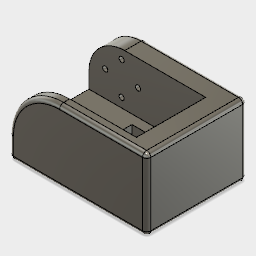
top_bracket (Autodesk Fusion 360 design; units mm, degrees)
Autodesk Fusion 360 part; units mm, degrees
sketch "Sketch1" plane through (0, 0, 0) normal (0, 1, 0) x (1, 0, 0)
  line L0 (0, 0) -> (50, 0)
  line L1 (50, 0) -> (50, -31.77)
  line L2 (50, -31.77) -> (0, -31.77)
  line L3 (0, -31.77) -> (0, 0)
  line L4 (0, 0) -> (0, -15.885)
  line L5 (0, -15.885) -> (0, -9.635)
  line L6 (0, -15.885) -> (0, -22.135)
  line L7 (0, -22.135) -> (3.4, -22.135)
  line L8 (0, -9.635) -> (3.4, -9.635)
  circle A0 centre (3.4, -9.635) radius 1
  circle A1 centre (3.4, -22.135) radius 1
  line L9 (0, -15.885) -> (0, -7.885)
  line L10 (0, -15.885) -> (0, -23.885)
  line L11 (0, -7.885) -> (17, -7.885)
  line L12 (0, -23.885) -> (17, -23.885)
  circle A2 centre (17, -23.885) radius 1
  circle A3 centre (17, -7.885) radius 1
  line L13 (0, -15.885) -> (10.8, -15.885)
  circle A4 centre (10.8, -15.885) radius 5.375
  line L14 (0, -23.885) -> (33, -23.885)
  line L15 (0, -7.885) -> (33, -7.885)
  circle A5 centre (33, -7.885) radius 1
  circle A6 centre (33, -23.885) radius 1
  line L16 (0, -15.885) -> (43.5, -15.885)
  line L17 (43.5, -15.885) -> (43.5, -25.885)
  line L18 (43.5, -15.885) -> (43.5, -5.885)
  line L19 (43.5, -5.885) -> (36.36, -5.885)
  line L20 (43.5, -25.885) -> (36.36, -25.885)
  line L21 (36.36, -25.885) -> (36.36, -19.885)
  line L22 (36.36, -5.885) -> (36.36, -11.885)
  line L23 (36.36, -11.885) -> (43.5, -11.885)
  line L24 (36.36, -19.885) -> (43.5, -19.885)
  line L25 (0, -15.885) -> (24, -15.885)
  line L26 (24, -15.885) -> (31, -15.885)
  line L27 (31, -15.885) -> (31.5, -15.885)
  line L28 (24, -15.885) -> (24, -3.885)
  line L29 (31.5, -15.885) -> (31.5, -3.885)
  line L30 (31.5, -15.885) -> (31.5, -27.885)
  line L31 (24, -15.885) -> (24, -27.885)
  line L32 (31.5, -3.885) -> (24, -3.885)
  line L33 (24, -27.885) -> (31.5, -27.885)
  line L34 (24, -27.885) -> (22, -27.885)
  line L35 (22, -27.885) -> (22, -3.885)
  line L36 (22, -3.885) -> (24, -3.885)
  dimension "d1" = 50
  dimension "d2" = 31.77
  dimension "d3" = 6.25
  dimension "d4" = 6.25
  dimension "d5" = 3.4
  dimension "d6" = 3.4
  dimension "d7" = 2
  dimension "d8" = 2
  dimension "d9" = 8
  dimension "d10" = 8
  dimension "d11" = 17
  dimension "d12" = 17
  dimension "d13" = 2
  dimension "d14" = 2
  dimension "d15" = 10.8
  dimension "d16" = 10.75
  dimension "d17" = 33
  dimension "d18" = 33
  dimension "d19" = 2
  dimension "d20" = 2
  dimension "d21" = 43.5
  dimension "d22" = 10
  dimension "d23" = 10
  dimension "d24" = 7.14
  dimension "d25" = 7.14
  dimension "d26" = 6
  dimension "d27" = 6
  dimension "d28" = 24
  dimension "d29" = 7
  dimension "d30" = 0.5
  dimension "d31" = 12
  dimension "d32" = 12
  dimension "d33" = 12
  dimension "d34" = 12
  dimension "d35" = 2
  dimension "d36" = 24
  constraint horizontal L0
  constraint vertical L1
  constraint horizontal L2
  constraint vertical L3
  constraint coincident L0.start L3.end
  constraint midpoint L3
  constraint horizontal L11
  constraint vertical L17
  constraint vertical L18
  constraint vertical L22
  constraint coincident L18
  constraint perpendicular L18 L23
  constraint coincident L17 L0.start
  constraint perpendicular L17 L24
  constraint perpendicular L28 L32
  constraint perpendicular L30 L33
  constraint perpendicular L31 L34
  constraint perpendicular L28 L36
  measures "d2" distance of L0.start
  measures "d3" distance of L0.start
  measures "d7" diameter of A0
  measures "d8" diameter of A1
  measures "d9" distance of L0.start
  measures "d13" diameter of A2
  measures "d14" diameter of A3
  measures "d16" diameter of A4
  measures "d19" diameter of A5
  measures "d20" diameter of A6
  measures "d23" distance of L0.start
  measures "d26" distance of L0.start
  measures "d27" distance of L0.start
  measures "d33" distance of L0.start
  measures "d34" distance of L0.start
  measures "d36" distance of L0.start
extrude "Extrude1" add sketch "Sketch1" along normal blind 3 contours L0 L1 L2 L3 L4 L11 L12 A2 A3 L14 L15 L29 L30 L32 L33 L34 L35 L36 | L3 L4 L5 L9 L11 A3 L13 A4 L15 L16 L25 L35 | L3 L6 L10 L12 A2 L13 A4 L14 L16 L25 L35
extrude "Extrude2" add sketch "Sketch1" along normal blind 7 contours L13 A4 L16 L25 | L13 A4 L16 L25 | L17 L20 L21 L24 | L18 L19 L22 L23
extrude "Extrude3" add 1 faces at (44.6337, 0, 13.363) along direction (0, -1, 0) blind 7
extrude "Extrude4" cut 3 faces at (38.74, 7, 21.885) (41.12, 7, 9.885) (11.9171, 7, 13.428) along direction (0, -1, 0) blind 8
sketch "Sketch2" plane through (0, 3, 0) normal (0, 1, 0) x (-1, 0, 0)
  circle A0 centre (-33, 7.885) radius 1
  line L0 (-43.5, 11.885) -> (-36.36, 11.885)
  line L1 (-36.36, 11.885) -> (-36.36, 5.885)
  line L2 (-36.36, 5.885) -> (-43.5, 5.885)
  line L3 (-43.5, 5.885) -> (-43.5, 11.885)
  circle A1 centre (-33, 23.885) radius 1
  line L4 (-36.36, 25.885) -> (-36.36, 19.885)
  line L5 (-36.36, 19.885) -> (-43.5, 19.885)
  line L6 (-43.5, 19.885) -> (-43.5, 25.885)
  line L7 (-43.5, 25.885) -> (-36.36, 25.885)
  circle A2 centre (-3.4, 22.135) radius 1
  circle A3 centre (-17, 23.885) radius 1
  circle A4 centre (-17, 7.885) radius 1
  circle A5 centre (-3.4, 9.635) radius 1
  circle A6 centre (-10.8, 15.885) radius 5.375
  line L8 (-31.5, 27.885) -> (-22, 27.885)
  line L9 (-22, 27.885) -> (-22, 3.885)
  line L10 (-22, 3.885) -> (-31.5, 3.885)
  line L11 (-31.5, 3.885) -> (-31.5, 27.885)
  line L12 (0, 0) -> (0, 31.77)
  line L13 (0, 31.77) -> (-50, 31.77)
  line L14 (-50, 31.77) -> (-50, 0)
  line L15 (-50, 0) -> (0, 0)
  line L16 (-20.4906, 2.4501) -> (-32.562, 2.4501)
  line L17 (-32.562, 2.4501) -> (-32.562, 29.6236)
  line L18 (-32.562, 29.6236) -> (-20.4906, 29.6236)
  line L19 (-20.4906, 29.6236) -> (-20.4906, 2.4501)
  circle A7 centre (-10.8, 15.885) radius 5.75
  line L20 (-36, 5.5) -> (-44, 5.5)
  line L21 (-44, 5.5) -> (-44, 12.5)
  line L22 (-44, 12.5) -> (-36, 12.5)
  line L23 (-36, 12.5) -> (-36, 5.5)
  line L24 (-36, 19.5) -> (-43.8348, 19.5)
  line L25 (-43.8348, 19.5) -> (-43.8348, 26.2715)
  line L26 (-43.8348, 26.2715) -> (-36, 26.2715)
  line L27 (-36, 26.2715) -> (-36, 19.5)
  circle A8 centre (-33, 23.885) radius 1.25
  circle A9 centre (-33, 7.885) radius 1.25
  circle A10 centre (-17, 7.885) radius 1.25
  circle A11 centre (-17, 23.885) radius 1.25
  circle A12 centre (-3.4, 22.135) radius 1.25
  circle A13 centre (-3.4, 9.635) radius 1.25
  dimension "d45" = 11.5
  dimension "d46" = 2.5
  dimension "d47" = 2.5
  dimension "d48" = 2.5
  dimension "d49" = 2.5
  dimension "d50" = 2.5
  dimension "d51" = 2.5
  constraint horizontal L16
  constraint vertical L17
  constraint horizontal L18
  constraint vertical L19
  constraint concentric A6 A7
  constraint horizontal L20
  constraint vertical L21
  constraint horizontal L22
  constraint vertical L23
  constraint horizontal L24
  constraint vertical L25
  constraint horizontal L26
  constraint vertical L27
  constraint concentric A1 A8
  constraint concentric A0 A9
  constraint concentric A4 A10
  constraint concentric A3 A11
  constraint concentric A2 A12
  constraint concentric A5 A13
  measures "d45" diameter of A7
  measures "d46" diameter of A8
  measures "d47" diameter of A9
  measures "d48" diameter of A10
  measures "d49" diameter of A11
  measures "d50" diameter of A12
  measures "d51" diameter of A13
extrude "Extrude5" cut sketch "Sketch2" against normal blind 4 contours A7 | L20 L21 L22 L23 | L24 L25 L26 L27
extrude "Extrude6" cut sketch "Sketch2" against normal blind 11 contours A0 L17 A9 | A0 L17 A9 | L16 L17 L18 L19 A8 A9 | A1 L17 A8 | A1 L17 A8 | A10 | A11 | A12 | A13
extrude "Extrude7" add 1 faces at (16.6667, -0.3333, 0) along direction (0, 0, -1) blind 12
sketch "Sketch3" plane through (0, 3, 0) normal (0, 1, 0) x (-1, 0, 0)
  circle A0 centre (-3.4, 9.635) radius 1.25
  circle A1 centre (-17, 7.885) radius 1.25
  circle A2 centre (-3.4, 22.135) radius 1.25
  circle A3 centre (-17, 23.885) radius 1.25
  line L0 (-32.562, 9.0557) -> (-32.562, 22.7143)
  arc A4 (-32.562, 25.0557) -> (-32.562, 22.7143) centre (-33, 23.885) ccw
  line L1 (-32.562, 25.0557) -> (-32.562, 29.6236)
  line L2 (-32.562, 29.6236) -> (-20.4906, 29.6236)
  line L3 (-20.4906, 29.6236) -> (-20.4906, 2.4501)
  line L4 (-20.4906, 2.4501) -> (-32.562, 2.4501)
  line L5 (-32.562, 2.4501) -> (-32.562, 6.7143)
  arc A5 (-32.562, 9.0557) -> (-32.562, 6.7143) centre (-33, 7.885) ccw
  circle A6 centre (-10.8, 15.885) radius 5.75
  line L6 (-44, 5.5) -> (-44, 12.5)
  line L7 (-44, 12.5) -> (-36, 12.5)
  line L8 (-36, 12.5) -> (-36, 5.5)
  line L9 (-36, 5.5) -> (-44, 5.5)
  line L10 (-43.8348, 19.5) -> (-43.8348, 26.2715)
  line L11 (-43.8348, 26.2715) -> (-36, 26.2715)
  line L12 (-36, 26.2715) -> (-36, 19.5)
  line L13 (-36, 19.5) -> (-43.8348, 19.5)
  line L14 (0, -12) -> (0, 31.77)
  line L15 (0, 31.77) -> (-50, 31.77)
  line L16 (-50, 31.77) -> (-50, -12)
  line L17 (-50, -12) -> (0, -12)
  line L18 (0, -12) -> (-50, -12)
  line L19 (-50, -12) -> (-50, -2)
  line L20 (-50, -2) -> (0, -2)
  line L21 (0, -2) -> (0, -12)
  dimension "d58" = 10
  constraint horizontal L18
  constraint vertical L19
  constraint horizontal L20
  constraint vertical L21
extrude "Extrude8" add sketch "Sketch3" along normal blind 25 contours L14 L16 L17 L18 L19 L20 L21
extrude "Extrude9" add 1 faces at (50, -3.6667, 5.9233) along direction (1, 0, 0) blind 12
sketch "Sketch4" plane through (0, 3, 0) normal (0, 1, 0) x (-1, 0, 0)
  line L0 (-62, -2) -> (0, -2)
  line L1 (0, -2) -> (0, 31.77)
  line L2 (0, 31.77) -> (-62, 31.77)
  line L3 (-62, 31.77) -> (-62, -2)
  line L4 (-43.8348, 19.5) -> (-43.8348, 26.2715)
  line L5 (-43.8348, 26.2715) -> (-36, 26.2715)
  line L6 (-36, 26.2715) -> (-36, 19.5)
  line L7 (-36, 19.5) -> (-43.8348, 19.5)
  line L8 (-44, 5.5) -> (-44, 12.5)
  line L9 (-44, 12.5) -> (-36, 12.5)
  line L10 (-36, 12.5) -> (-36, 5.5)
  line L11 (-36, 5.5) -> (-44, 5.5)
  circle A0 centre (-10.8, 15.885) radius 5.75
  line L12 (-32.562, 9.0557) -> (-32.562, 22.7143)
  arc A1 (-32.562, 25.0557) -> (-32.562, 22.7143) centre (-33, 23.885) ccw
  line L13 (-32.562, 25.0557) -> (-32.562, 29.6236)
  line L14 (-32.562, 29.6236) -> (-20.4906, 29.6236)
  line L15 (-20.4906, 29.6236) -> (-20.4906, 2.4501)
  line L16 (-20.4906, 2.4501) -> (-32.562, 2.4501)
  line L17 (-32.562, 2.4501) -> (-32.562, 6.7143)
  arc A2 (-32.562, 9.0557) -> (-32.562, 6.7143) centre (-33, 7.885) ccw
  circle A3 centre (-17, 23.885) radius 1.25
  circle A4 centre (-3.4, 22.135) radius 1.25
  circle A5 centre (-17, 7.885) radius 1.25
  circle A6 centre (-3.4, 9.635) radius 1.25
  line L18 (-62, 31.77) -> (-52, 31.77)
  line L19 (-52, 31.77) -> (-52, -2)
  line L20 (-52, -2) -> (-62, -2)
  line L21 (-62, -2) -> (-62, 31.77)
  dimension "d63" = 10
  constraint horizontal L18
  constraint vertical L19
  constraint horizontal L20
  constraint vertical L21
extrude "Extrude10" add sketch "Sketch4" along normal blind 25 contours L0 L2 L3 L18 L19 L20 L21
sketch "Sketch5" plane through (0, 0, -2) normal (0, 0, 1) x (1, 0, 0)
  line L0 (52, 3) -> (52, 28)
  line L1 (52, 28) -> (0, 28)
  line L2 (0, 28) -> (0, 3)
  line L3 (0, 3) -> (52, 3)
  line L4 (0, 28) -> (3, 28)
  line L5 (3, 28) -> (3, 15.5)
  line L6 (3, 15.5) -> (11, 15.5)
  line L7 (11, 15.5) -> (11, 23.5)
  line L8 (11, 15.5) -> (11, 7.5)
  line L9 (11, 15.5) -> (19, 15.5)
  circle A0 centre (19, 15.5) radius 1.25
  circle A1 centre (11, 23.5) radius 1.25
  circle A2 centre (11, 7.5) radius 1.25
  circle A3 centre (3, 15.5) radius 1.25
  dimension "d66" = 3
  dimension "d67" = 12.5
  dimension "d68" = 8
  dimension "d69" = 8
  dimension "d70" = 8
  dimension "d71" = 8
  dimension "d72" = 2.5
  dimension "d73" = 2.5
  dimension "d74" = 2.5
  dimension "d75" = 2.5
  constraint coincident L1
  constraint perpendicular L2 L4
  constraint perpendicular L5 L6
  measures "d72" diameter of A0
  measures "d73" diameter of A1
  measures "d74" diameter of A2
  measures "d75" diameter of A3
extrude "Extrude11" cut sketch "Sketch5" against normal blind 23 contours L5 L6 A3 | L5 L6 A3 | A0 | A1 | A2
extrude "Extrude12" cut 1 faces at (52.7454, -7, 9.2799) along direction (0, 1, 0) blind 6
sketch "Sketch6" plane through (0, -1, 0) normal (0, -1, 0) x (1, 0, 0)
  circle A0 centre (10.8, 15.885) radius 5.75
  line L0 (44, 12.5) -> (44, 5.5)
  line L1 (44, 5.5) -> (36, 5.5)
  line L2 (36, 5.5) -> (36, 12.5)
  line L3 (36, 12.5) -> (44, 12.5)
  line L4 (43.8348, 26.2715) -> (43.8348, 19.5)
  line L5 (43.8348, 19.5) -> (36, 19.5)
  line L6 (36, 19.5) -> (36, 26.2715)
  line L7 (36, 26.2715) -> (43.8348, 26.2715)
  circle A1 centre (3.4, 9.635) radius 1.25
  circle A2 centre (17, 7.885) radius 1.25
  circle A3 centre (3.4, 22.135) radius 1.25
  circle A4 centre (17, 23.885) radius 1.25
  line L8 (32.562, 22.7143) -> (32.562, 9.0557)
  arc A5 (32.562, 6.7143) -> (32.562, 9.0557) centre (33, 7.885) ccw
  line L9 (32.562, 6.7143) -> (32.562, 2.4501)
  line L10 (32.562, 2.4501) -> (20.4906, 2.4501)
  line L11 (20.4906, 2.4501) -> (20.4906, 29.6236)
  line L12 (20.4906, 29.6236) -> (32.562, 29.6236)
  line L13 (32.562, 29.6236) -> (32.562, 25.0557)
  arc A6 (32.562, 22.7143) -> (32.562, 25.0557) centre (33, 23.885) ccw
  line L14 (0, 31.77) -> (0, -12)
  line L15 (0, -12) -> (62, -12)
  line L16 (62, -12) -> (62, 31.77)
  line L17 (62, 31.77) -> (0, 31.77)
  circle A7 centre (3.4, 9.635) radius 2.5
  circle A8 centre (3.4, 22.135) radius 2.5
  circle A9 centre (17, 23.885) radius 2.5
  circle A10 centre (17, 7.885) radius 2.5
  circle A11 centre (33, 7.885) radius 2.5
  circle A12 centre (33, 23.885) radius 2.5
  dimension "d80" = 5
  dimension "d81" = 5
  dimension "d82" = 5
  dimension "d83" = 5
  dimension "d84" = 5
  dimension "d85" = 5
  constraint concentric A1 A7
  constraint concentric A3 A8
  constraint concentric A4 A9
  constraint concentric A2 A10
  constraint concentric A5 A11
  constraint concentric A6 A12
  measures "d80" diameter of A7
  measures "d81" diameter of A8
  measures "d82" diameter of A9
  measures "d83" diameter of A10
  measures "d84" diameter of A11
  measures "d85" diameter of A12
extrude "Extrude13" cut sketch "Sketch6" against normal blind 2 contours L8 L13 A6 A12 | L8 A5 L9 A11 | A7 | A8 | A9 | A10 picked at (32.803, 21.8157) picked at (32.803, 5.8157)
extrude "Extrude14" add 1 faces at (58.6667, 10, 31.77) along direction (0, 0, 1) blind 5
sketch "Sketch7" plane through (0, 3, 0) normal (0, 1, 0) x (-1, 0, 0)
  circle A0 centre (-3.4, 9.635) radius 1.25
  circle A1 centre (-17, 7.885) radius 1.25
  circle A2 centre (-3.4, 22.135) radius 1.25
  circle A3 centre (-17, 23.885) radius 1.25
  line L0 (-32.562, 9.0557) -> (-32.562, 22.7143)
  arc A4 (-32.562, 25.0557) -> (-32.562, 22.7143) centre (-33, 23.885) ccw
  line L1 (-32.562, 25.0557) -> (-32.562, 29.6236)
  line L2 (-32.562, 29.6236) -> (-20.4906, 29.6236)
  line L3 (-20.4906, 29.6236) -> (-20.4906, 2.4501)
  line L4 (-20.4906, 2.4501) -> (-32.562, 2.4501)
  line L5 (-32.562, 2.4501) -> (-32.562, 6.7143)
  arc A5 (-32.562, 9.0557) -> (-32.562, 6.7143) centre (-33, 7.885) ccw
  circle A6 centre (-10.8, 15.885) radius 5.75
  line L6 (-44, 5.5) -> (-44, 12.5)
  line L7 (-44, 12.5) -> (-36, 12.5)
  line L8 (-36, 12.5) -> (-36, 5.5)
  line L9 (-36, 5.5) -> (-44, 5.5)
  line L10 (-43.8348, 19.5) -> (-43.8348, 26.2715)
  line L11 (-43.8348, 26.2715) -> (-36, 26.2715)
  line L12 (-36, 26.2715) -> (-36, 19.5)
  line L13 (-36, 19.5) -> (-43.8348, 19.5)
  line L14 (-52, 36.77) -> (-52, -2)
  line L15 (-52, -2) -> (0, -2)
  line L16 (0, -2) -> (0, 36.77)
  line L17 (0, 36.77) -> (-52, 36.77)
  line L18 (-52, 36.77) -> (0, 36.77)
  line L19 (0, 36.77) -> (0, 31.77)
  line L20 (0, 31.77) -> (-52, 31.77)
  line L21 (-52, 31.77) -> (-52, 36.77)
  dimension "d90" = 52
  dimension "d91" = 5
  constraint horizontal L18
  constraint vertical L19
  constraint horizontal L20
  constraint vertical L21
extrude "Extrude15" add sketch "Sketch7" along normal blind 25 contours L14 L16 L17 L18 L19 L20 L21
extrude "Extrude16" add 1 faces at (0, 10, -8.6667) along direction (-1, 0, 0) blind 5
extrude "Extrude17" add 6 faces at (19.0694, 1, 23.6987) (5.474, 1, 22.0108) (5.4694, 1, 9.4487) (19.0694, 1, 7.6987) (32.803, 1, 25.9543) (32.803, 1, 9.9543) along direction (0, -1, 0) blind 2
extrude "Extrude18" add 1 faces at (56, -1, 12.4233) along direction (0, -1, 0) blind 6
fillet "Fillet6" radius 17.5 1 edges at (-5, 28, -7)
fillet "Fillet7" radius 24.5 1 edges at (-5, 28, 34.27)
fillet "Fillet8" radius 2 3 edges at (40.75, 28, 36.77) (2.1759, 20.8241, 36.77) (-5, -1.75, 36.77)
fillet "Fillet9" radius 2 3 edges at (37.25, 28, -12) (0.1256, 22.8744, -12) (-5, 1.75, -12)
fillet "Fillet10" radius 2 5 edges at (62, 9.5, -12) (62, 27.4142, -11.4142) (62, 28, 12.385) (62, 27.4142, 36.1842) (62, 9.5, 36.77)
fillet "Fillet11" radius 2 8 edges at (61.4142, -7, -11.4142) (62, -7, 12.385) (61.4142, -7, 36.1842) (28.5, -7, 36.77) (-4.4142, -7, 36.1842) (-5, -7, 12.385) (-4.4142, -7, -11.4142) (28.5, -7, -12)
